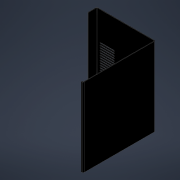
# Autodesk Inventor part: PlateAMP
Saved by Autodesk Inventor 2022 (Build 260153070, 153G)
## iProperties
Created: 2021-12-15
Part Number: PlateAMP
Material: Типовые
Document SubType Name: Sheet Metal
Designer: kalugin_a
Density: 1 g/cm^3
Flat Pattern Width: 21.7 cm
Flat Pattern Length: 38.4179 cm
Flat Pattern Area: 833.668 cm^2
Sheet Metal Rule: По умолчанию_мм
Sheet Metal Width: 217,000 мм
Sheet Metal Length: 384,179 мм
Sheet Metal Area: 83366,791 мм^2
Appearance: По умолчанию
Author: kalugin_a
Autodesk Inventor part; units mm, degrees
ref_plane "YZ Plane" through (0, 0, 0) normal (1, 0, 0) x (0, 1, 0)
ref_plane "XZ Plane" through (0, 0, 0) normal (0, 1, 0) x (-1, 0, 0)
ref_plane "XY Plane" through (0, 0, 0) normal (0, 0, 1) x (1, 0, 0)
sketch "Эскиз1" plane through (0, 0, 0) normal (0, 0, 1) x (1, 0, 0)
  line L0 (0, 0) -> (162, 0)
  line L1 (162, 0) -> (162, 217)
  line L2 (162, 217) -> (0, 217)
  line L3 (0, 217) -> (0, 0)
  line L4 (152.9674, 23.6384) -> (92.9674, 23.6384) construction
  line L5 (151.4674, 25.1384) -> (94.4674, 25.1384)
  line L6 (94.4674, 22.1384) -> (151.4674, 22.1384)
  arc A0 (151.4674, 22.1384) -> (151.4674, 25.1384) centre (151.4674, 23.6384) ccw
  arc A1 (94.4674, 25.1384) -> (94.4674, 22.1384) centre (94.4674, 23.6384) ccw
  line L7 (152.9674, 29.6384) -> (92.9674, 29.6384) construction
  line L8 (151.4674, 31.1384) -> (94.4674, 31.1384)
  line L9 (94.4674, 28.1384) -> (151.4674, 28.1384)
  arc A2 (151.4674, 28.1384) -> (151.4674, 31.1384) centre (151.4674, 29.6384) ccw
  arc A3 (94.4674, 31.1384) -> (94.4674, 28.1384) centre (94.4674, 29.6384) ccw
  line L10 (152.9674, 35.6384) -> (92.9674, 35.6384) construction
  line L11 (151.4674, 37.1384) -> (94.4674, 37.1384)
  line L12 (94.4674, 34.1384) -> (151.4674, 34.1384)
  arc A4 (151.4674, 34.1384) -> (151.4674, 37.1384) centre (151.4674, 35.6384) ccw
  arc A5 (94.4674, 37.1384) -> (94.4674, 34.1384) centre (94.4674, 35.6384) ccw
  line L13 (152.9674, 41.6384) -> (92.9674, 41.6384) construction
  line L14 (151.4674, 43.1384) -> (94.4674, 43.1384)
  line L15 (94.4674, 40.1384) -> (151.4674, 40.1384)
  arc A6 (151.4674, 40.1384) -> (151.4674, 43.1384) centre (151.4674, 41.6384) ccw
  arc A7 (94.4674, 43.1384) -> (94.4674, 40.1384) centre (94.4674, 41.6384) ccw
  line L16 (152.9674, 47.6384) -> (92.9674, 47.6384) construction
  line L17 (151.4674, 49.1384) -> (94.4674, 49.1384)
  line L18 (94.4674, 46.1384) -> (151.4674, 46.1384)
  arc A8 (151.4674, 46.1384) -> (151.4674, 49.1384) centre (151.4674, 47.6384) ccw
  arc A9 (94.4674, 49.1384) -> (94.4674, 46.1384) centre (94.4674, 47.6384) ccw
  line L19 (152.9674, 53.6384) -> (92.9674, 53.6384) construction
  line L20 (151.4674, 55.1384) -> (94.4674, 55.1384)
  line L21 (94.4674, 52.1384) -> (151.4674, 52.1384)
  arc A10 (151.4674, 52.1384) -> (151.4674, 55.1384) centre (151.4674, 53.6384) ccw
  arc A11 (94.4674, 55.1384) -> (94.4674, 52.1384) centre (94.4674, 53.6384) ccw
  line L22 (152.9674, 59.6384) -> (92.9674, 59.6384) construction
  line L23 (151.4674, 61.1384) -> (94.4674, 61.1384)
  line L24 (94.4674, 58.1384) -> (151.4674, 58.1384)
  arc A12 (151.4674, 58.1384) -> (151.4674, 61.1384) centre (151.4674, 59.6384) ccw
  arc A13 (94.4674, 61.1384) -> (94.4674, 58.1384) centre (94.4674, 59.6384) ccw
  line L25 (152.9674, 65.6384) -> (92.9674, 65.6384) construction
  line L26 (151.4674, 67.1384) -> (94.4674, 67.1384)
  line L27 (94.4674, 64.1384) -> (151.4674, 64.1384)
  arc A14 (151.4674, 64.1384) -> (151.4674, 67.1384) centre (151.4674, 65.6384) ccw
  arc A15 (94.4674, 67.1384) -> (94.4674, 64.1384) centre (94.4674, 65.6384) ccw
  line L28 (152.9674, 71.6384) -> (92.9674, 71.6384) construction
  line L29 (151.4674, 73.1384) -> (94.4674, 73.1384)
  line L30 (94.4674, 70.1384) -> (151.4674, 70.1384)
  arc A16 (151.4674, 70.1384) -> (151.4674, 73.1384) centre (151.4674, 71.6384) ccw
  arc A17 (94.4674, 73.1384) -> (94.4674, 70.1384) centre (94.4674, 71.6384) ccw
  line L31 (152.9674, 77.6384) -> (92.9674, 77.6384) construction
  line L32 (151.4674, 79.1384) -> (94.4674, 79.1384)
  line L33 (94.4674, 76.1384) -> (151.4674, 76.1384)
  arc A18 (151.4674, 76.1384) -> (151.4674, 79.1384) centre (151.4674, 77.6384) ccw
  arc A19 (94.4674, 79.1384) -> (94.4674, 76.1384) centre (94.4674, 77.6384) ccw
  line L34 (152.9674, 83.6384) -> (92.9674, 83.6384) construction
  line L35 (151.4674, 85.1384) -> (94.4674, 85.1384)
  line L36 (94.4674, 82.1384) -> (151.4674, 82.1384)
  arc A20 (151.4674, 82.1384) -> (151.4674, 85.1384) centre (151.4674, 83.6384) ccw
  arc A21 (94.4674, 85.1384) -> (94.4674, 82.1384) centre (94.4674, 83.6384) ccw
  line L37 (152.9674, 89.6384) -> (92.9674, 89.6384) construction
  line L38 (151.4674, 91.1384) -> (94.4674, 91.1384)
  line L39 (94.4674, 88.1384) -> (151.4674, 88.1384)
  arc A22 (151.4674, 88.1384) -> (151.4674, 91.1384) centre (151.4674, 89.6384) ccw
  arc A23 (94.4674, 91.1384) -> (94.4674, 88.1384) centre (94.4674, 89.6384) ccw
  line L40 (152.9674, 95.6384) -> (92.9674, 95.6384) construction
  line L41 (151.4674, 97.1384) -> (94.4674, 97.1384)
  line L42 (94.4674, 94.1384) -> (151.4674, 94.1384)
  arc A24 (151.4674, 94.1384) -> (151.4674, 97.1384) centre (151.4674, 95.6384) ccw
  arc A25 (94.4674, 97.1384) -> (94.4674, 94.1384) centre (94.4674, 95.6384) ccw
  line L43 (152.9674, 101.6384) -> (92.9674, 101.6384) construction
  line L44 (151.4674, 103.1384) -> (94.4674, 103.1384)
  line L45 (94.4674, 100.1384) -> (151.4674, 100.1384)
  arc A26 (151.4674, 100.1384) -> (151.4674, 103.1384) centre (151.4674, 101.6384) ccw
  arc A27 (94.4674, 103.1384) -> (94.4674, 100.1384) centre (94.4674, 101.6384) ccw
  line L46 (152.9674, 107.6384) -> (92.9674, 107.6384) construction
  line L47 (151.4674, 109.1384) -> (94.4674, 109.1384)
  line L48 (94.4674, 106.1384) -> (151.4674, 106.1384)
  arc A28 (151.4674, 106.1384) -> (151.4674, 109.1384) centre (151.4674, 107.6384) ccw
  arc A29 (94.4674, 109.1384) -> (94.4674, 106.1384) centre (94.4674, 107.6384) ccw
  line L49 (152.9674, 113.6384) -> (92.9674, 113.6384) construction
  line L50 (151.4674, 115.1384) -> (94.4674, 115.1384)
  line L51 (94.4674, 112.1384) -> (151.4674, 112.1384)
  arc A30 (151.4674, 112.1384) -> (151.4674, 115.1384) centre (151.4674, 113.6384) ccw
  arc A31 (94.4674, 115.1384) -> (94.4674, 112.1384) centre (94.4674, 113.6384) ccw
  line L52 (152.9674, 119.6384) -> (92.9674, 119.6384) construction
  line L53 (151.4674, 121.1384) -> (94.4674, 121.1384)
  line L54 (94.4674, 118.1384) -> (151.4674, 118.1384)
  arc A32 (151.4674, 118.1384) -> (151.4674, 121.1384) centre (151.4674, 119.6384) ccw
  arc A33 (94.4674, 121.1384) -> (94.4674, 118.1384) centre (94.4674, 119.6384) ccw
  line L55 (152.9674, 125.6384) -> (92.9674, 125.6384) construction
  line L56 (151.4674, 127.1384) -> (94.4674, 127.1384)
  line L57 (94.4674, 124.1384) -> (151.4674, 124.1384)
  arc A34 (151.4674, 124.1384) -> (151.4674, 127.1384) centre (151.4674, 125.6384) ccw
  arc A35 (94.4674, 127.1384) -> (94.4674, 124.1384) centre (94.4674, 125.6384) ccw
  line L58 (152.9674, 131.6384) -> (92.9674, 131.6384) construction
  line L59 (151.4674, 133.1384) -> (94.4674, 133.1384)
  line L60 (94.4674, 130.1384) -> (151.4674, 130.1384)
  arc A36 (151.4674, 130.1384) -> (151.4674, 133.1384) centre (151.4674, 131.6384) ccw
  arc A37 (94.4674, 133.1384) -> (94.4674, 130.1384) centre (94.4674, 131.6384) ccw
  line L61 (152.9674, 137.6384) -> (92.9674, 137.6384) construction
  line L62 (151.4674, 139.1384) -> (94.4674, 139.1384)
  line L63 (94.4674, 136.1384) -> (151.4674, 136.1384)
  arc A38 (151.4674, 136.1384) -> (151.4674, 139.1384) centre (151.4674, 137.6384) ccw
  arc A39 (94.4674, 139.1384) -> (94.4674, 136.1384) centre (94.4674, 137.6384) ccw
  line L64 (152.9674, 143.6384) -> (92.9674, 143.6384) construction
  line L65 (151.4674, 145.1384) -> (94.4674, 145.1384)
  line L66 (94.4674, 142.1384) -> (151.4674, 142.1384)
  arc A40 (151.4674, 142.1384) -> (151.4674, 145.1384) centre (151.4674, 143.6384) ccw
  arc A41 (94.4674, 145.1384) -> (94.4674, 142.1384) centre (94.4674, 143.6384) ccw
  line L67 (152.9674, 149.6384) -> (92.9674, 149.6384) construction
  line L68 (151.4674, 151.1384) -> (94.4674, 151.1384)
  line L69 (94.4674, 148.1384) -> (151.4674, 148.1384)
  arc A42 (151.4674, 148.1384) -> (151.4674, 151.1384) centre (151.4674, 149.6384) ccw
  arc A43 (94.4674, 151.1384) -> (94.4674, 148.1384) centre (94.4674, 149.6384) ccw
  line L70 (152.9674, 155.6384) -> (92.9674, 155.6384) construction
  line L71 (151.4674, 157.1384) -> (94.4674, 157.1384)
  line L72 (94.4674, 154.1384) -> (151.4674, 154.1384)
  arc A44 (151.4674, 154.1384) -> (151.4674, 157.1384) centre (151.4674, 155.6384) ccw
  arc A45 (94.4674, 157.1384) -> (94.4674, 154.1384) centre (94.4674, 155.6384) ccw
  line L73 (152.9674, 161.6384) -> (92.9674, 161.6384) construction
  line L74 (151.4674, 163.1384) -> (94.4674, 163.1384)
  line L75 (94.4674, 160.1384) -> (151.4674, 160.1384)
  arc A46 (151.4674, 160.1384) -> (151.4674, 163.1384) centre (151.4674, 161.6384) ccw
  arc A47 (94.4674, 163.1384) -> (94.4674, 160.1384) centre (94.4674, 161.6384) ccw
  line L76 (22.9674, 23.6384) -> (-37.0326, 23.6384) construction
  line L77 (21.4674, 25.1384) -> (-35.5326, 25.1384)
  line L78 (-35.5326, 22.1384) -> (21.4674, 22.1384)
  arc A48 (21.4674, 22.1384) -> (21.4674, 25.1384) centre (21.4674, 23.6384) ccw
  arc A49 (-35.5326, 25.1384) -> (-35.5326, 22.1384) centre (-35.5326, 23.6384) ccw
  line L79 (22.9674, 29.6384) -> (-37.0326, 29.6384) construction
  line L80 (21.4674, 31.1384) -> (-35.5326, 31.1384)
  line L81 (-35.5326, 28.1384) -> (21.4674, 28.1384)
  arc A50 (21.4674, 28.1384) -> (21.4674, 31.1384) centre (21.4674, 29.6384) ccw
  arc A51 (-35.5326, 31.1384) -> (-35.5326, 28.1384) centre (-35.5326, 29.6384) ccw
  line L82 (22.9674, 35.6384) -> (-37.0326, 35.6384) construction
  line L83 (21.4674, 37.1384) -> (-35.5326, 37.1384)
  line L84 (-35.5326, 34.1384) -> (21.4674, 34.1384)
  arc A52 (21.4674, 34.1384) -> (21.4674, 37.1384) centre (21.4674, 35.6384) ccw
  arc A53 (-35.5326, 37.1384) -> (-35.5326, 34.1384) centre (-35.5326, 35.6384) ccw
  line L85 (22.9674, 41.6384) -> (-37.0326, 41.6384) construction
  line L86 (21.4674, 43.1384) -> (-35.5326, 43.1384)
  line L87 (-35.5326, 40.1384) -> (21.4674, 40.1384)
  arc A54 (21.4674, 40.1384) -> (21.4674, 43.1384) centre (21.4674, 41.6384) ccw
  arc A55 (-35.5326, 43.1384) -> (-35.5326, 40.1384) centre (-35.5326, 41.6384) ccw
  line L88 (22.9674, 47.6384) -> (-37.0326, 47.6384) construction
  line L89 (21.4674, 49.1384) -> (-35.5326, 49.1384)
  line L90 (-35.5326, 46.1384) -> (21.4674, 46.1384)
  arc A56 (21.4674, 46.1384) -> (21.4674, 49.1384) centre (21.4674, 47.6384) ccw
  arc A57 (-35.5326, 49.1384) -> (-35.5326, 46.1384) centre (-35.5326, 47.6384) ccw
  line L91 (22.9674, 53.6384) -> (-37.0326, 53.6384) construction
  line L92 (21.4674, 55.1384) -> (-35.5326, 55.1384)
  line L93 (-35.5326, 52.1384) -> (21.4674, 52.1384)
  arc A58 (21.4674, 52.1384) -> (21.4674, 55.1384) centre (21.4674, 53.6384) ccw
  arc A59 (-35.5326, 55.1384) -> (-35.5326, 52.1384) centre (-35.5326, 53.6384) ccw
  line L94 (22.9674, 59.6384) -> (-37.0326, 59.6384) construction
  line L95 (21.4674, 61.1384) -> (-35.5326, 61.1384)
  line L96 (-35.5326, 58.1384) -> (21.4674, 58.1384)
  arc A60 (21.4674, 58.1384) -> (21.4674, 61.1384) centre (21.4674, 59.6384) ccw
  arc A61 (-35.5326, 61.1384) -> (-35.5326, 58.1384) centre (-35.5326, 59.6384) ccw
  line L97 (22.9674, 65.6384) -> (-37.0326, 65.6384) construction
  line L98 (21.4674, 67.1384) -> (-35.5326, 67.1384)
  line L99 (-35.5326, 64.1384) -> (21.4674, 64.1384)
  arc A62 (21.4674, 64.1384) -> (21.4674, 67.1384) centre (21.4674, 65.6384) ccw
  arc A63 (-35.5326, 67.1384) -> (-35.5326, 64.1384) centre (-35.5326, 65.6384) ccw
  line L100 (22.9674, 71.6384) -> (-37.0326, 71.6384) construction
  line L101 (21.4674, 73.1384) -> (-35.5326, 73.1384)
  line L102 (-35.5326, 70.1384) -> (21.4674, 70.1384)
  arc A64 (21.4674, 70.1384) -> (21.4674, 73.1384) centre (21.4674, 71.6384) ccw
  arc A65 (-35.5326, 73.1384) -> (-35.5326, 70.1384) centre (-35.5326, 71.6384) ccw
  line L103 (22.9674, 77.6384) -> (-37.0326, 77.6384) construction
  line L104 (21.4674, 79.1384) -> (-35.5326, 79.1384)
  line L105 (-35.5326, 76.1384) -> (21.4674, 76.1384)
  arc A66 (21.4674, 76.1384) -> (21.4674, 79.1384) centre (21.4674, 77.6384) ccw
  arc A67 (-35.5326, 79.1384) -> (-35.5326, 76.1384) centre (-35.5326, 77.6384) ccw
  line L106 (22.9674, 83.6384) -> (-37.0326, 83.6384) construction
  line L107 (21.4674, 85.1384) -> (-35.5326, 85.1384)
  line L108 (-35.5326, 82.1384) -> (21.4674, 82.1384)
  arc A68 (21.4674, 82.1384) -> (21.4674, 85.1384) centre (21.4674, 83.6384) ccw
  arc A69 (-35.5326, 85.1384) -> (-35.5326, 82.1384) centre (-35.5326, 83.6384) ccw
  line L109 (22.9674, 89.6384) -> (-37.0326, 89.6384) construction
  line L110 (21.4674, 91.1384) -> (-35.5326, 91.1384)
  line L111 (-35.5326, 88.1384) -> (21.4674, 88.1384)
  arc A70 (21.4674, 88.1384) -> (21.4674, 91.1384) centre (21.4674, 89.6384) ccw
  arc A71 (-35.5326, 91.1384) -> (-35.5326, 88.1384) centre (-35.5326, 89.6384) ccw
  line L112 (22.9674, 95.6384) -> (-37.0326, 95.6384) construction
  line L113 (21.4674, 97.1384) -> (-35.5326, 97.1384)
  line L114 (-35.5326, 94.1384) -> (21.4674, 94.1384)
  arc A72 (21.4674, 94.1384) -> (21.4674, 97.1384) centre (21.4674, 95.6384) ccw
  arc A73 (-35.5326, 97.1384) -> (-35.5326, 94.1384) centre (-35.5326, 95.6384) ccw
  line L115 (22.9674, 101.6384) -> (-37.0326, 101.6384) construction
  line L116 (21.4674, 103.1384) -> (-35.5326, 103.1384)
  line L117 (-35.5326, 100.1384) -> (21.4674, 100.1384)
  arc A74 (21.4674, 100.1384) -> (21.4674, 103.1384) centre (21.4674, 101.6384) ccw
  arc A75 (-35.5326, 103.1384) -> (-35.5326, 100.1384) centre (-35.5326, 101.6384) ccw
  line L118 (22.9674, 107.6384) -> (-37.0326, 107.6384) construction
  line L119 (21.4674, 109.1384) -> (-35.5326, 109.1384)
  line L120 (-35.5326, 106.1384) -> (21.4674, 106.1384)
  arc A76 (21.4674, 106.1384) -> (21.4674, 109.1384) centre (21.4674, 107.6384) ccw
  arc A77 (-35.5326, 109.1384) -> (-35.5326, 106.1384) centre (-35.5326, 107.6384) ccw
  line L121 (22.9674, 113.6384) -> (-37.0326, 113.6384) construction
  line L122 (21.4674, 115.1384) -> (-35.5326, 115.1384)
  line L123 (-35.5326, 112.1384) -> (21.4674, 112.1384)
  arc A78 (21.4674, 112.1384) -> (21.4674, 115.1384) centre (21.4674, 113.6384) ccw
  arc A79 (-35.5326, 115.1384) -> (-35.5326, 112.1384) centre (-35.5326, 113.6384) ccw
  line L124 (22.9674, 119.6384) -> (-37.0326, 119.6384) construction
  line L125 (21.4674, 121.1384) -> (-35.5326, 121.1384)
  line L126 (-35.5326, 118.1384) -> (21.4674, 118.1384)
  arc A80 (21.4674, 118.1384) -> (21.4674, 121.1384) centre (21.4674, 119.6384) ccw
  arc A81 (-35.5326, 121.1384) -> (-35.5326, 118.1384) centre (-35.5326, 119.6384) ccw
  line L127 (22.9674, 125.6384) -> (-37.0326, 125.6384) construction
  line L128 (21.4674, 127.1384) -> (-35.5326, 127.1384)
  line L129 (-35.5326, 124.1384) -> (21.4674, 124.1384)
  arc A82 (21.4674, 124.1384) -> (21.4674, 127.1384) centre (21.4674, 125.6384) ccw
  arc A83 (-35.5326, 127.1384) -> (-35.5326, 124.1384) centre (-35.5326, 125.6384) ccw
  line L130 (22.9674, 131.6384) -> (-37.0326, 131.6384) construction
  line L131 (21.4674, 133.1384) -> (-35.5326, 133.1384)
  line L132 (-35.5326, 130.1384) -> (21.4674, 130.1384)
  arc A84 (21.4674, 130.1384) -> (21.4674, 133.1384) centre (21.4674, 131.6384) ccw
  arc A85 (-35.5326, 133.1384) -> (-35.5326, 130.1384) centre (-35.5326, 131.6384) ccw
  line L133 (22.9674, 137.6384) -> (-37.0326, 137.6384) construction
  line L134 (21.4674, 139.1384) -> (-35.5326, 139.1384)
  line L135 (-35.5326, 136.1384) -> (21.4674, 136.1384)
  arc A86 (21.4674, 136.1384) -> (21.4674, 139.1384) centre (21.4674, 137.6384) ccw
  arc A87 (-35.5326, 139.1384) -> (-35.5326, 136.1384) centre (-35.5326, 137.6384) ccw
  line L136 (22.9674, 143.6384) -> (-37.0326, 143.6384) construction
  line L137 (21.4674, 145.1384) -> (-35.5326, 145.1384)
  line L138 (-35.5326, 142.1384) -> (21.4674, 142.1384)
  arc A88 (21.4674, 142.1384) -> (21.4674, 145.1384) centre (21.4674, 143.6384) ccw
  arc A89 (-35.5326, 145.1384) -> (-35.5326, 142.1384) centre (-35.5326, 143.6384) ccw
  line L139 (22.9674, 149.6384) -> (-37.0326, 149.6384) construction
  line L140 (21.4674, 151.1384) -> (-35.5326, 151.1384)
  line L141 (-35.5326, 148.1384) -> (21.4674, 148.1384)
  arc A90 (21.4674, 148.1384) -> (21.4674, 151.1384) centre (21.4674, 149.6384) ccw
  arc A91 (-35.5326, 151.1384) -> (-35.5326, 148.1384) centre (-35.5326, 149.6384) ccw
  line L142 (22.9674, 155.6384) -> (-37.0326, 155.6384) construction
  line L143 (21.4674, 157.1384) -> (-35.5326, 157.1384)
  line L144 (-35.5326, 154.1384) -> (21.4674, 154.1384)
  arc A92 (21.4674, 154.1384) -> (21.4674, 157.1384) centre (21.4674, 155.6384) ccw
  arc A93 (-35.5326, 157.1384) -> (-35.5326, 154.1384) centre (-35.5326, 155.6384) ccw
  line L145 (22.9674, 161.6384) -> (-37.0326, 161.6384) construction
  line L146 (21.4674, 163.1384) -> (-35.5326, 163.1384)
  line L147 (-35.5326, 160.1384) -> (21.4674, 160.1384)
  arc A94 (21.4674, 160.1384) -> (21.4674, 163.1384) centre (21.4674, 161.6384) ccw
  arc A95 (-35.5326, 163.1384) -> (-35.5326, 160.1384) centre (-35.5326, 161.6384) ccw
  point P0 (122.9674, 23.6384)
  point P1 (122.9674, 29.6384)
  point P2 (122.9674, 35.6384)
  point P3 (122.9674, 41.6384)
  point P4 (122.9674, 47.6384)
  point P5 (122.9674, 53.6384)
  point P6 (122.9674, 59.6384)
  point P7 (122.9674, 65.6384)
  point P8 (122.9674, 71.6384)
  point P9 (122.9674, 77.6384)
  point P10 (122.9674, 83.6384)
  point P11 (122.9674, 89.6384)
  point P12 (122.9674, 95.6384)
  point P13 (122.9674, 101.6384)
  point P14 (122.9674, 107.6384)
  point P15 (122.9674, 113.6384)
  point P16 (122.9674, 119.6384)
  point P17 (122.9674, 125.6384)
  point P18 (122.9674, 131.6384)
  point P19 (122.9674, 137.6384)
  point P20 (122.9674, 143.6384)
  point P21 (122.9674, 149.6384)
  point P22 (122.9674, 155.6384)
  point P23 (122.9674, 161.6384)
  point P24 (-7.0326, 23.6384)
  point P25 (-7.0326, 29.6384)
  point P26 (-7.0326, 35.6384)
  point P27 (-7.0326, 41.6384)
  point P28 (-7.0326, 47.6384)
  point P29 (-7.0326, 53.6384)
  point P30 (-7.0326, 59.6384)
  point P31 (-7.0326, 65.6384)
  point P32 (-7.0326, 71.6384)
  point P33 (-7.0326, 77.6384)
  point P34 (-7.0326, 83.6384)
  point P35 (-7.0326, 89.6384)
  point P36 (-7.0326, 95.6384)
  point P37 (-7.0326, 101.6384)
  point P38 (-7.0326, 107.6384)
  point P39 (-7.0326, 113.6384)
  point P40 (-7.0326, 119.6384)
  point P41 (-7.0326, 125.6384)
  point P42 (-7.0326, 131.6384)
  point P43 (-7.0326, 137.6384)
  point P44 (-7.0326, 143.6384)
  point P45 (-7.0326, 149.6384)
  point P46 (-7.0326, 155.6384)
  point P47 (-7.0326, 161.6384)
  dimension "d11" = 217
  dimension "d12" = 162
  dimension "d33" = 60
  dimension "d34" = 3
  dimension "d50" = 6
  dimension "d53" = 130
  constraints: 392 end point, 288 point on circle, 96 centre point, 96 point on line, 4 tangent, 3 parallel, 2 horizontal, 2 perpendicular, 1 midpoint, 1 vertical, 658 other
  measures "d11" distance of L0.end L1.end
  measures "d12" distance of L1.end L2.end
  measures "d33" distance of L4.start L4.end
  measures "d34" diameter of A1
  measures "d50" distance of L5.start L8.start
  measures "d53" distance of L5.start L77.start
extrude "Пластина1" add sketch "Эскиз1" against normal blind 1.5 contours L3 L78 A48 L77 L81 A50 L80 L84 A52 L83 L87 A54 L86 L90 A56 L89 L93 A58 L92 L96 A60 L95 L99 A62 L98 L102 A64 L101 L105 A66 L104 L108 A68 L107 L111 A70 L110 L114 A72 L113 L117 A74 L116 L120 A76 L119 L123 A78 L122 L126 A80 L125 L129 A82 L128 L132 A84 L131 L135 A86 L134 L138 A88 L137 L141 A90 L140 L144 A92 L143 L147 A94 L146 L2 L1 L0 | L3 L77 A48 L78 | L3 L80 A50 L81 | L146 A94 L147 L3 | L3 L83 A52 L84 | L143 A92 L144 L3 | L3 L86 A54 L87 | L140 A90 L141 L3 | L3 L89 A56 L90 | L137 A88 L138 L3 | L3 L92 A58 L93 | L134 A86 L135 L3 | L3 L95 A60 L96 | L131 A84 L132 L3 | L3 L98 A62 L99 | L128 A82 L129 L3 | L3 L101 A64 L102 | L125 A80 L126 L3 | L3 L104 A66 L105 | L122 A78 L123 L3 | L3 L107 A68 L108 | L119 A76 L120 L3 | L3 L110 A70 L111 | L116 A74 L117 L3 | L3 L113 A72 L114 | A0 L6 A1 L5 | A2 L9 A3 L8 | A4 L12 A5 L11 | A6 L15 A7 L14 | A8 L18 A9 L17 | A10 L21 A11 L20 | A12 L24 A13 L23 | A14 L27 A15 L26 | A16 L30 A17 L29 | A18 L33 A19 L32 | A20 L36 A21 L35 | A22 L39 A23 L38 | A24 L42 A25 L41 | A26 L45 A27 L44 | A28 L48 A29 L47 | A30 L51 A31 L50 | A32 L54 A33 L53 | A34 L57 A35 L56 | A36 L60 A37 L59 | A38 L63 A39 L62 | A40 L66 A41 L65 | A42 L69 A43 L68 | A44 L72 A45 L71 | A46 L75 A47 L74
sketch "Эскиз2" plane through (1.5, 0, -1.5) normal (-1, 0, 0) x (0, -1, 0)
  line L0 (-217, 0) -> (0, 0)
  line L1 (0, 0) -> (0, 25)
  line L2 (0, 25) -> (-217, 25)
  line L3 (-217, 25) -> (-217, 0)
  constraints: 6 end point, 1 horizontal, 1 perpendicular, 1 vertical
edge flange "Фланец1" height 25 angle 90 thickness 1.5 bend radius 1.5 thickness toward (-1, 0, 0) relief straight relief width 1.5 relief depth 0.75 edges at (0, 108.5, 0) wall of the first edge with corners at (1.5, 217, -1.5) (1.5, 0, -1.5) (1.5, 0, 23.5) (1.5, 217, 23.5)
bend "Сгиб1"
corner "УглСтык1"
sketch "Эскиз3" plane through (160.5, 217, -1.5) normal (1, 0, 0) x (0, 1, 0)
  line L0 (-217, 0) -> (0, 0)
  line L1 (0, 0) -> (0, 200)
  line L2 (0, 200) -> (-217, 200)
  line L3 (-217, 200) -> (-217, 0)
  constraints: 6 end point, 1 horizontal, 1 perpendicular, 1 vertical
edge flange "Фланец2" height 200 angle 90 thickness 1.5 bend radius 1.5 thickness toward (1, 0, 0) relief straight relief width 1.5 relief depth 0.75 edges at (162, 108.5, 0) wall of the first edge with corners at (160.5, 0, -1.5) (160.5, 217, -1.5) (160.5, 217, 198.5) (160.5, 0, 198.5)
bend "Сгиб2"
corner "УглСтык2"
sketch "Эскиз4" plane through (162, 0, 197) normal (0, 0, 1) x (-1, 0, 0)
  line L0 (0, 217) -> (0, 0)
  line L1 (0, 0) -> (5, 0)
  line L2 (5, 0) -> (5, 217)
  line L3 (5, 217) -> (0, 217)
  constraints: 6 end point, 1 horizontal, 1 perpendicular, 1 vertical
edge flange "Фланец3" height 5 angle 90 thickness 1.5 bend radius 1.5 thickness toward (0, 0, 1) relief straight relief width 1.5 relief depth 0.75 edges at (162, 108.5, 198.5) wall of the first edge with corners at (162, 217, 197) (162, 0, 197) (157, 0, 197) (157, 217, 197)
bend "Сгиб3"
corner "УглСтык3"
sketch "Эскиз5" plane through (0, 0, -1.5) normal (0, 0, -1) x (-1, 0, 0)
  line L0 (-245.4892, 265.8375) -> (-245.4892, 0.8375)
  line L1 (-150, 137) -> (-110, 137) construction
  line L2 (-148.5, 135.5) -> (-111.5, 135.5)
  line L3 (-111.5, 138.5) -> (-148.5, 138.5)
  arc A0 (-148.5, 138.5) -> (-148.5, 135.5) centre (-148.5, 137) ccw
  arc A1 (-111.5, 135.5) -> (-111.5, 138.5) centre (-111.5, 137) ccw
  line L4 (-159, 217) -> (-3, 217) projected
  line L5 (-150, 131) -> (-110, 131) construction
  line L6 (-148.5, 129.5) -> (-111.5, 129.5)
  line L7 (-111.5, 132.5) -> (-148.5, 132.5)
  arc A2 (-148.5, 132.5) -> (-148.5, 129.5) centre (-148.5, 131) ccw
  arc A3 (-111.5, 129.5) -> (-111.5, 132.5) centre (-111.5, 131) ccw
  line L8 (-150, 125) -> (-110, 125) construction
  line L9 (-148.5, 123.5) -> (-111.5, 123.5)
  line L10 (-111.5, 126.5) -> (-148.5, 126.5)
  arc A4 (-148.5, 126.5) -> (-148.5, 123.5) centre (-148.5, 125) ccw
  arc A5 (-111.5, 123.5) -> (-111.5, 126.5) centre (-111.5, 125) ccw
  line L11 (-150, 119) -> (-110, 119) construction
  line L12 (-148.5, 117.5) -> (-111.5, 117.5)
  line L13 (-111.5, 120.5) -> (-148.5, 120.5)
  arc A6 (-148.5, 120.5) -> (-148.5, 117.5) centre (-148.5, 119) ccw
  arc A7 (-111.5, 117.5) -> (-111.5, 120.5) centre (-111.5, 119) ccw
  line L14 (-150, 113) -> (-110, 113) construction
  line L15 (-148.5, 111.5) -> (-111.5, 111.5)
  line L16 (-111.5, 114.5) -> (-148.5, 114.5)
  arc A8 (-148.5, 114.5) -> (-148.5, 111.5) centre (-148.5, 113) ccw
  arc A9 (-111.5, 111.5) -> (-111.5, 114.5) centre (-111.5, 113) ccw
  line L17 (-150, 107) -> (-110, 107) construction
  line L18 (-148.5, 105.5) -> (-111.5, 105.5)
  line L19 (-111.5, 108.5) -> (-148.5, 108.5)
  arc A10 (-148.5, 108.5) -> (-148.5, 105.5) centre (-148.5, 107) ccw
  arc A11 (-111.5, 105.5) -> (-111.5, 108.5) centre (-111.5, 107) ccw
  line L20 (-150, 101) -> (-110, 101) construction
  line L21 (-148.5, 99.5) -> (-111.5, 99.5)
  line L22 (-111.5, 102.5) -> (-148.5, 102.5)
  arc A12 (-148.5, 102.5) -> (-148.5, 99.5) centre (-148.5, 101) ccw
  arc A13 (-111.5, 99.5) -> (-111.5, 102.5) centre (-111.5, 101) ccw
  line L23 (-150, 95) -> (-110, 95) construction
  line L24 (-148.5, 93.5) -> (-111.5, 93.5)
  line L25 (-111.5, 96.5) -> (-148.5, 96.5)
  arc A14 (-148.5, 96.5) -> (-148.5, 93.5) centre (-148.5, 95) ccw
  arc A15 (-111.5, 93.5) -> (-111.5, 96.5) centre (-111.5, 95) ccw
  line L26 (-150, 89) -> (-110, 89) construction
  line L27 (-148.5, 87.5) -> (-111.5, 87.5)
  line L28 (-111.5, 90.5) -> (-148.5, 90.5)
  arc A16 (-148.5, 90.5) -> (-148.5, 87.5) centre (-148.5, 89) ccw
  arc A17 (-111.5, 87.5) -> (-111.5, 90.5) centre (-111.5, 89) ccw
  line L29 (-150, 83) -> (-110, 83) construction
  line L30 (-148.5, 81.5) -> (-111.5, 81.5)
  line L31 (-111.5, 84.5) -> (-148.5, 84.5)
  arc A18 (-148.5, 84.5) -> (-148.5, 81.5) centre (-148.5, 83) ccw
  arc A19 (-111.5, 81.5) -> (-111.5, 84.5) centre (-111.5, 83) ccw
  line L32 (-150, 77) -> (-110, 77) construction
  line L33 (-148.5, 75.5) -> (-111.5, 75.5)
  line L34 (-111.5, 78.5) -> (-148.5, 78.5)
  arc A20 (-148.5, 78.5) -> (-148.5, 75.5) centre (-148.5, 77) ccw
  arc A21 (-111.5, 75.5) -> (-111.5, 78.5) centre (-111.5, 77) ccw
  line L35 (-150, 71) -> (-110, 71) construction
  line L36 (-148.5, 69.5) -> (-111.5, 69.5)
  line L37 (-111.5, 72.5) -> (-148.5, 72.5)
  arc A22 (-148.5, 72.5) -> (-148.5, 69.5) centre (-148.5, 71) ccw
  arc A23 (-111.5, 69.5) -> (-111.5, 72.5) centre (-111.5, 71) ccw
  line L38 (-150, 65) -> (-110, 65) construction
  line L39 (-148.5, 63.5) -> (-111.5, 63.5)
  line L40 (-111.5, 66.5) -> (-148.5, 66.5)
  arc A24 (-148.5, 66.5) -> (-148.5, 63.5) centre (-148.5, 65) ccw
  arc A25 (-111.5, 63.5) -> (-111.5, 66.5) centre (-111.5, 65) ccw
  line L41 (-150, 59) -> (-110, 59) construction
  line L42 (-148.5, 57.5) -> (-111.5, 57.5)
  line L43 (-111.5, 60.5) -> (-148.5, 60.5)
  arc A26 (-148.5, 60.5) -> (-148.5, 57.5) centre (-148.5, 59) ccw
  arc A27 (-111.5, 57.5) -> (-111.5, 60.5) centre (-111.5, 59) ccw
  line L44 (-150, 53) -> (-110, 53) construction
  line L45 (-148.5, 51.5) -> (-111.5, 51.5)
  line L46 (-111.5, 54.5) -> (-148.5, 54.5)
  arc A28 (-148.5, 54.5) -> (-148.5, 51.5) centre (-148.5, 53) ccw
  arc A29 (-111.5, 51.5) -> (-111.5, 54.5) centre (-111.5, 53) ccw
  line L47 (-150, 47) -> (-110, 47) construction
  line L48 (-148.5, 45.5) -> (-111.5, 45.5)
  line L49 (-111.5, 48.5) -> (-148.5, 48.5)
  arc A30 (-148.5, 48.5) -> (-148.5, 45.5) centre (-148.5, 47) ccw
  arc A31 (-111.5, 45.5) -> (-111.5, 48.5) centre (-111.5, 47) ccw
  line L50 (-150, 41) -> (-110, 41) construction
  line L51 (-148.5, 39.5) -> (-111.5, 39.5)
  line L52 (-111.5, 42.5) -> (-148.5, 42.5)
  arc A32 (-148.5, 42.5) -> (-148.5, 39.5) centre (-148.5, 41) ccw
  arc A33 (-111.5, 39.5) -> (-111.5, 42.5) centre (-111.5, 41) ccw
  line L53 (-150, 35) -> (-110, 35) construction
  line L54 (-148.5, 33.5) -> (-111.5, 33.5)
  line L55 (-111.5, 36.5) -> (-148.5, 36.5)
  arc A34 (-148.5, 36.5) -> (-148.5, 33.5) centre (-148.5, 35) ccw
  arc A35 (-111.5, 33.5) -> (-111.5, 36.5) centre (-111.5, 35) ccw
  line L56 (-150, 29) -> (-110, 29) construction
  line L57 (-148.5, 27.5) -> (-111.5, 27.5)
  line L58 (-111.5, 30.5) -> (-148.5, 30.5)
  arc A36 (-148.5, 30.5) -> (-148.5, 27.5) centre (-148.5, 29) ccw
  arc A37 (-111.5, 27.5) -> (-111.5, 30.5) centre (-111.5, 29) ccw
  line L59 (-150, 23) -> (-110, 23) construction
  line L60 (-148.5, 21.5) -> (-111.5, 21.5)
  line L61 (-111.5, 24.5) -> (-148.5, 24.5)
  arc A38 (-148.5, 24.5) -> (-148.5, 21.5) centre (-148.5, 23) ccw
  arc A39 (-111.5, 21.5) -> (-111.5, 24.5) centre (-111.5, 23) ccw
  line L62 (-150, 17) -> (-110, 17) construction
  line L63 (-148.5, 15.5) -> (-111.5, 15.5)
  line L64 (-111.5, 18.5) -> (-148.5, 18.5)
  arc A40 (-148.5, 18.5) -> (-148.5, 15.5) centre (-148.5, 17) ccw
  arc A41 (-111.5, 15.5) -> (-111.5, 18.5) centre (-111.5, 17) ccw
  line L65 (-150, 11) -> (-110, 11) construction
  line L66 (-148.5, 9.5) -> (-111.5, 9.5)
  line L67 (-111.5, 12.5) -> (-148.5, 12.5)
  arc A42 (-148.5, 12.5) -> (-148.5, 9.5) centre (-148.5, 11) ccw
  arc A43 (-111.5, 9.5) -> (-111.5, 12.5) centre (-111.5, 11) ccw
  line L68 (-50, 137) -> (-10, 137) construction
  line L69 (-48.5, 135.5) -> (-11.5, 135.5)
  line L70 (-11.5, 138.5) -> (-48.5, 138.5)
  arc A44 (-48.5, 138.5) -> (-48.5, 135.5) centre (-48.5, 137) ccw
  arc A45 (-11.5, 135.5) -> (-11.5, 138.5) centre (-11.5, 137) ccw
  line L71 (-50, 131) -> (-10, 131) construction
  line L72 (-48.5, 129.5) -> (-11.5, 129.5)
  line L73 (-11.5, 132.5) -> (-48.5, 132.5)
  arc A46 (-48.5, 132.5) -> (-48.5, 129.5) centre (-48.5, 131) ccw
  arc A47 (-11.5, 129.5) -> (-11.5, 132.5) centre (-11.5, 131) ccw
  line L74 (-50, 125) -> (-10, 125) construction
  line L75 (-48.5, 123.5) -> (-11.5, 123.5)
  line L76 (-11.5, 126.5) -> (-48.5, 126.5)
  arc A48 (-48.5, 126.5) -> (-48.5, 123.5) centre (-48.5, 125) ccw
  arc A49 (-11.5, 123.5) -> (-11.5, 126.5) centre (-11.5, 125) ccw
  line L77 (-50, 119) -> (-10, 119) construction
  line L78 (-48.5, 117.5) -> (-11.5, 117.5)
  line L79 (-11.5, 120.5) -> (-48.5, 120.5)
  arc A50 (-48.5, 120.5) -> (-48.5, 117.5) centre (-48.5, 119) ccw
  arc A51 (-11.5, 117.5) -> (-11.5, 120.5) centre (-11.5, 119) ccw
  line L80 (-50, 113) -> (-10, 113) construction
  line L81 (-48.5, 111.5) -> (-11.5, 111.5)
  line L82 (-11.5, 114.5) -> (-48.5, 114.5)
  arc A52 (-48.5, 114.5) -> (-48.5, 111.5) centre (-48.5, 113) ccw
  arc A53 (-11.5, 111.5) -> (-11.5, 114.5) centre (-11.5, 113) ccw
  line L83 (-50, 107) -> (-10, 107) construction
  line L84 (-48.5, 105.5) -> (-11.5, 105.5)
  line L85 (-11.5, 108.5) -> (-48.5, 108.5)
  arc A54 (-48.5, 108.5) -> (-48.5, 105.5) centre (-48.5, 107) ccw
  arc A55 (-11.5, 105.5) -> (-11.5, 108.5) centre (-11.5, 107) ccw
  line L86 (-50, 101) -> (-10, 101) construction
  line L87 (-48.5, 99.5) -> (-11.5, 99.5)
  line L88 (-11.5, 102.5) -> (-48.5, 102.5)
  arc A56 (-48.5, 102.5) -> (-48.5, 99.5) centre (-48.5, 101) ccw
  arc A57 (-11.5, 99.5) -> (-11.5, 102.5) centre (-11.5, 101) ccw
  line L89 (-50, 95) -> (-10, 95) construction
  line L90 (-48.5, 93.5) -> (-11.5, 93.5)
  line L91 (-11.5, 96.5) -> (-48.5, 96.5)
  arc A58 (-48.5, 96.5) -> (-48.5, 93.5) centre (-48.5, 95) ccw
  arc A59 (-11.5, 93.5) -> (-11.5, 96.5) centre (-11.5, 95) ccw
  line L92 (-50, 89) -> (-10, 89) construction
  line L93 (-48.5, 87.5) -> (-11.5, 87.5)
  line L94 (-11.5, 90.5) -> (-48.5, 90.5)
  arc A60 (-48.5, 90.5) -> (-48.5, 87.5) centre (-48.5, 89) ccw
  arc A61 (-11.5, 87.5) -> (-11.5, 90.5) centre (-11.5, 89) ccw
  line L95 (-50, 83) -> (-10, 83) construction
  line L96 (-48.5, 81.5) -> (-11.5, 81.5)
  line L97 (-11.5, 84.5) -> (-48.5, 84.5)
  arc A62 (-48.5, 84.5) -> (-48.5, 81.5) centre (-48.5, 83) ccw
  arc A63 (-11.5, 81.5) -> (-11.5, 84.5) centre (-11.5, 83) ccw
  line L98 (-50, 77) -> (-10, 77) construction
  line L99 (-48.5, 75.5) -> (-11.5, 75.5)
  line L100 (-11.5, 78.5) -> (-48.5, 78.5)
  arc A64 (-48.5, 78.5) -> (-48.5, 75.5) centre (-48.5, 77) ccw
  arc A65 (-11.5, 75.5) -> (-11.5, 78.5) centre (-11.5, 77) ccw
  line L101 (-50, 71) -> (-10, 71) construction
  line L102 (-48.5, 69.5) -> (-11.5, 69.5)
  line L103 (-11.5, 72.5) -> (-48.5, 72.5)
  arc A66 (-48.5, 72.5) -> (-48.5, 69.5) centre (-48.5, 71) ccw
  arc A67 (-11.5, 69.5) -> (-11.5, 72.5) centre (-11.5, 71) ccw
  line L104 (-50, 65) -> (-10, 65) construction
  line L105 (-48.5, 63.5) -> (-11.5, 63.5)
  line L106 (-11.5, 66.5) -> (-48.5, 66.5)
  arc A68 (-48.5, 66.5) -> (-48.5, 63.5) centre (-48.5, 65) ccw
  arc A69 (-11.5, 63.5) -> (-11.5, 66.5) centre (-11.5, 65) ccw
  line L107 (-50, 59) -> (-10, 59) construction
  line L108 (-48.5, 57.5) -> (-11.5, 57.5)
  line L109 (-11.5, 60.5) -> (-48.5, 60.5)
  arc A70 (-48.5, 60.5) -> (-48.5, 57.5) centre (-48.5, 59) ccw
  arc A71 (-11.5, 57.5) -> (-11.5, 60.5) centre (-11.5, 59) ccw
  line L110 (-50, 53) -> (-10, 53) construction
  line L111 (-48.5, 51.5) -> (-11.5, 51.5)
  line L112 (-11.5, 54.5) -> (-48.5, 54.5)
  arc A72 (-48.5, 54.5) -> (-48.5, 51.5) centre (-48.5, 53) ccw
  arc A73 (-11.5, 51.5) -> (-11.5, 54.5) centre (-11.5, 53) ccw
  line L113 (-50, 47) -> (-10, 47) construction
  line L114 (-48.5, 45.5) -> (-11.5, 45.5)
  line L115 (-11.5, 48.5) -> (-48.5, 48.5)
  arc A74 (-48.5, 48.5) -> (-48.5, 45.5) centre (-48.5, 47) ccw
  arc A75 (-11.5, 45.5) -> (-11.5, 48.5) centre (-11.5, 47) ccw
  line L116 (-50, 41) -> (-10, 41) construction
  line L117 (-48.5, 39.5) -> (-11.5, 39.5)
  line L118 (-11.5, 42.5) -> (-48.5, 42.5)
  arc A76 (-48.5, 42.5) -> (-48.5, 39.5) centre (-48.5, 41) ccw
  arc A77 (-11.5, 39.5) -> (-11.5, 42.5) centre (-11.5, 41) ccw
  line L119 (-50, 35) -> (-10, 35) construction
  line L120 (-48.5, 33.5) -> (-11.5, 33.5)
  line L121 (-11.5, 36.5) -> (-48.5, 36.5)
  arc A78 (-48.5, 36.5) -> (-48.5, 33.5) centre (-48.5, 35) ccw
  arc A79 (-11.5, 33.5) -> (-11.5, 36.5) centre (-11.5, 35) ccw
  line L122 (-50, 29) -> (-10, 29) construction
  line L123 (-48.5, 27.5) -> (-11.5, 27.5)
  line L124 (-11.5, 30.5) -> (-48.5, 30.5)
  arc A80 (-48.5, 30.5) -> (-48.5, 27.5) centre (-48.5, 29) ccw
  arc A81 (-11.5, 27.5) -> (-11.5, 30.5) centre (-11.5, 29) ccw
  line L125 (-50, 23) -> (-10, 23) construction
  line L126 (-48.5, 21.5) -> (-11.5, 21.5)
  line L127 (-11.5, 24.5) -> (-48.5, 24.5)
  arc A82 (-48.5, 24.5) -> (-48.5, 21.5) centre (-48.5, 23) ccw
  arc A83 (-11.5, 21.5) -> (-11.5, 24.5) centre (-11.5, 23) ccw
  line L128 (-50, 17) -> (-10, 17) construction
  line L129 (-48.5, 15.5) -> (-11.5, 15.5)
  line L130 (-11.5, 18.5) -> (-48.5, 18.5)
  arc A84 (-48.5, 18.5) -> (-48.5, 15.5) centre (-48.5, 17) ccw
  arc A85 (-11.5, 15.5) -> (-11.5, 18.5) centre (-11.5, 17) ccw
  line L131 (-50, 11) -> (-10, 11) construction
  line L132 (-48.5, 9.5) -> (-11.5, 9.5)
  line L133 (-11.5, 12.5) -> (-48.5, 12.5)
  arc A86 (-48.5, 12.5) -> (-48.5, 9.5) centre (-48.5, 11) ccw
  arc A87 (-11.5, 9.5) -> (-11.5, 12.5) centre (-11.5, 11) ccw
  line L134 (0, 217) -> (0, 0) projected
  line L135 (-162, 0) -> (-162, 217) projected
  line L136 (-3, 0) -> (-159, 0) construction
  point P0 (-130, 137)
  point P1 (-130, 131)
  point P2 (-130, 125)
  point P3 (-130, 119)
  point P4 (-130, 113)
  point P5 (-130, 107)
  point P6 (-130, 101)
  point P7 (-130, 95)
  point P8 (-130, 89)
  point P9 (-130, 83)
  point P10 (-130, 77)
  point P11 (-130, 71)
  point P12 (-130, 65)
  point P13 (-130, 59)
  point P14 (-130, 53)
  point P15 (-130, 47)
  point P16 (-130, 41)
  point P17 (-130, 35)
  point P18 (-130, 29)
  point P19 (-130, 23)
  point P20 (-130, 17)
  point P21 (-130, 11)
  point P22 (-30, 137)
  point P23 (-30, 131)
  point P24 (-30, 125)
  point P25 (-30, 119)
  point P26 (-30, 113)
  point P27 (-30, 107)
  point P28 (-30, 101)
  point P29 (-30, 95)
  point P30 (-30, 89)
  point P31 (-30, 83)
  point P32 (-30, 77)
  point P33 (-30, 71)
  point P34 (-30, 65)
  point P35 (-30, 59)
  point P36 (-30, 53)
  point P37 (-30, 47)
  point P38 (-30, 41)
  point P39 (-30, 35)
  point P40 (-30, 29)
  point P41 (-30, 23)
  point P42 (-30, 17)
  point P43 (-30, 11)
  dimension "d35" = 40
  dimension "d36" = 3
  dimension "d56" = 80
  dimension "d60" = 6
  dimension "d63" = 100
  dimension "d69" = 12
  dimension "d70" = 10
  dimension "d71" = 6
  constraints: 354 end point, 264 point on circle, 88 centre point, 88 point on line, 4 tangent, 1 horizontal, 1 midpoint, 1 parallel, 1 vertical, 602 other
  measures "d35" distance of L1.start L1.end
  measures "d36" diameter of A1
  measures "d56" distance from line of L4 L1.end
  measures "d60" distance of L2.start L6.start
  measures "d63" distance of L2.start L69.start
  measures "d69" distance from line of L135 L5.start
  measures "d70" distance from line of L134 L68.end
  measures "d71" distance of A42.centre A40.centre
extrude "Вырез2" cut sketch "Эскиз5" against normal blind 1.5
equation "\"d73\" = Толщина"
equation "\"d0\" = Толщина"
equation "\"d1\" = Ширина_просечки"
equation "\"d2\" = Глубина_просечки"
equation "\"d3\" = Мин_остаток"
equation "\"d4\" = Радиус_перехода"
equation "\"d7\" = Радиус_гибки"
equation "\"d8\" = Размер_просечки"
equation "\"d9\" = Размер_зазора"
equation "\"d10\" = Радиус_Якоби"
equation "\"d13\" = Ширина_просечки"
equation "\"d14\" = Глубина_просечки"
equation "\"d15\" = Мин_остаток"
equation "\"d16\" = Радиус_перехода"
equation "\"d19\" = Радиус_гибки"
equation "\"d20\" = Размер_просечки"
equation "\"d21\" = Размер_зазора"
equation "\"d22\" = Радиус_Якоби"
equation "\"d23\" = Ширина_просечки"
equation "\"d24\" = Глубина_просечки"
equation "\"d25\" = Мин_остаток"
equation "\"d26\" = Радиус_перехода"
equation "\"d29\" = Радиус_гибки"
equation "\"d30\" = Размер_просечки"
equation "\"d31\" = Размер_зазора"
equation "\"d32\" = Радиус_Якоби"
equation "\"Радиус_гибки\" = Толщина"
equation "\"Ширина_просечки\" = Толщина"
equation "\"Глубина_просечки\" = 0.5 * Толщина"
equation "\"Размер_просечки\" = 4 * Толщина"
equation "\"Мин_остаток\" = 2 * Толщина"
equation "\"Радиус_перехода\" = Радиус_гибки"
equation "\"Радиус_Якоби\" = Радиус_гибки"
equation "\"Размер_зазора\" = Толщина"
equation "\"Толщина\" = 1.5"
